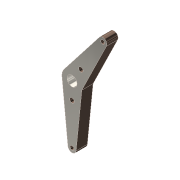
# Autodesk Inventor part: Lever
Saved by Autodesk Inventor 2022.2 (Build 262287010, 287A)
## iProperties
Created: 2022-12-22
Part Number: Lever
Material: Steel
Document SubType Name: Modeling
Designer: User
Mass: 98.2022 g
Surface Area: 55.5273 cm^2
Volume: 12.5098 cm^3
Density: 7.85 g/cm^3
Appearance: Gunmetal - Antique Polished
Author: User
Autodesk Inventor part; units mm, degrees
ref_plane "YZ Plane" through (0, 0, 0) normal (1, 0, 0) x (0, 1, 0)
ref_plane "XZ Plane" through (0, 0, 0) normal (0, 1, 0) x (-1, 0, 0)
ref_plane "XY Plane" through (0, 0, 0) normal (0, 0, 1) x (1, 0, 0)
sketch "Sketch1" plane through (0, 0, 0) normal (0, 0, 1) x (1, 0, 0)
  circle A0 centre (0, 0) radius 4.5
  line L0 (0, 0) -> (27.3538, 43.7752) construction
  line L1 (0, -76.1552) -> (0, 69.6997) construction
  line L2 (0, 0) -> (0, -51.6188) construction
  circle A1 centre (0, -51.6188) radius 1.7
  circle A2 centre (27.3538, 43.7752) radius 1.7
  arc A3 (30.6767, 42.1478) -> (24.4345, 46.0484) centre (27.3538, 43.7752) ccw
  arc A4 (-3.6804, -51.9996) -> (3.6804, -51.9996) centre (0, -51.6188) ccw
  line L3 (0, 0) -> (7.9488, 12.7207) construction
  circle A5 centre (7.9488, 12.7207) radius 2
  line L4 (0, 0) -> (0, -15) construction
  circle A6 centre (0, -15) radius 2
  line L5 (-7.1107, 5.5369) -> (24.4345, 46.0484)
  line L6 (-8.9644, -0.9275) -> (-3.6804, -51.9996)
  line L7 (8.7873, -2.6385) -> (30.6767, 42.1478)
  line L8 (8.7873, -2.6385) -> (3.6804, -51.9996)
  arc A7 (-7.1107, 5.5369) -> (-8.9644, -0.9275) centre (0, 0) ccw
  point P0 (8.0937, -3.9639)
  dimension "d0" = 9
  dimension "d2" = 32
  dimension "d3" = 51.6188
  dimension "d4" = 51.6188
  dimension "d5" = 3.4
  dimension "d6" = 3.4
  dimension "d7" = 3.7
  dimension "d8" = 3.7
  dimension "d9" = 15
  dimension "d10" = 4
  dimension "d11" = 15
  dimension "d12" = 4
  constraints: 16 end point, 8 centre point, 8 coincident, 6 point on circle, 4 tangent, 3 point on line, 3 symmetric about line
  measures "d0" diameter of A0
  measures "d2" angle of L0 L1
  measures "d3" distance of L0.start L0.end
  measures "d4" distance of L0.start L2.end
  measures "d5" diameter of A1
  measures "d6" diameter of A2
  measures "d7" radius of A3
  measures "d8" radius of A4
  measures "d9" distance of L0.start L3.end
  measures "d10" diameter of A5
  measures "d11" distance of L0.start L4.end
  measures "d12" diameter of A6
extrude "Extrusion1" add sketch "Sketch1" along normal blind 10
equation "\"d3\" = d4"
body "Solid1"
